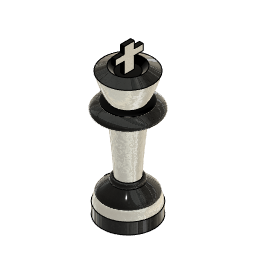
king_chess_piece (Autodesk Fusion 360 design; units mm, degrees)
Autodesk Fusion 360 part; units mm, degrees
sketch "Sketch2" plane through (0, 0, 0) normal (0, 1, 0) x (1, 0, 0)
  line L0 (0, 0) -> (-7, 0)
  line L1 (-7, 0) -> (-7, 3)
  spline S0 degree 5 poles (-7, 3) (-6.9874, 3.0714) (-6.9612, 3.2116) (-6.9188, 3.4141) (-6.856, 3.6679) (-6.7665, 3.9566) (-6.6647, 4.2138) (-6.5496, 4.4365) (-6.4202, 4.6222) (-6.2765, 4.7712) (-6.1194, 4.8856) (-5.9839, 4.9515) (-5.8769, 4.9875) (-5.8034, 5.0055) (-5.766, 5.013) knots 0 0 0 0 0 0 0.1 0.2 0.3 0.4 0.5 0.6 0.7 0.8 0.9 1 1 1 1 1 1
  spline S1 degree 5 poles (-5.766, 5.013) (-5.8491, 5.0166) (-6.0026, 5.0292) (-6.1954, 5.0646) (-6.376, 5.1453) (-6.4673, 5.3049) (-6.4171, 5.5264) (-6.2239, 5.8105) (-5.8977, 6.1528) (-5.4521, 6.5473) (-4.9009, 6.988) (-4.3843, 7.3737) (-3.9572, 7.6802) (-3.6553, 7.8921) (-3.5, 8) knots 0 0 0 0 0 0 0.1 0.2 0.3 0.4 0.5 0.6 0.7 0.8 0.9 1 1 1 1 1 1
  circle A0 centre (-2.9, 8.4) radius 0.7211
  spline S2 degree 5 poles (-2.8459, 9.1191) (-2.8432, 9.2564) (-2.8404, 9.5444) (-2.8435, 10.0169) (-2.8628, 10.7291) (-2.9134, 11.7639) (-2.9922, 12.9521) (-3.0997, 14.2974) (-3.2345, 15.791) (-3.3939, 17.4189) (-3.5752, 19.1663) (-3.736, 20.6501) (-3.8649, 21.8079) (-3.9544, 22.5994) (-4, 23) knots 0 0 0 0 0 0 0.1 0.2 0.3 0.4 0.5 0.6 0.7 0.8 0.9 1 1 1 1 1 1
  spline S3 degree 5 poles (-4, 23) (-4.2423, 23.0544) (-4.708, 23.1636) (-5.3496, 23.3289) (-6.0894, 23.5522) (-6.8078, 23.8366) (-7.2999, 24.1267) (-7.5451, 24.423) (-7.5279, 24.726) (-7.2529, 25.0355) (-6.737, 25.351) (-6.1462, 25.608) (-5.609, 25.8031) (-5.2099, 25.9342) (-5, 26) knots 0 0 0 0 0 0 0.1 0.2 0.3 0.4 0.5 0.6 0.7 0.8 0.9 1 1 1 1 1 1
  spline S4 degree 5 poles (-5, 26) (-5.0554, 26.027) (-5.1592, 26.0801) (-5.2942, 26.1566) (-5.432, 26.2523) (-5.5294, 26.3609) (-5.5464, 26.4575) (-5.4782, 26.5415) (-5.3253, 26.613) (-5.0938, 26.6728) (-4.7909, 26.722) (-4.4968, 26.7537) (-4.249, 26.7734) (-4.0719, 26.7848) (-3.9804, 26.7901) knots 0 0 0 0 0 0 0.1 0.2 0.3 0.4 0.5 0.6 0.7 0.8 0.9 1 1 1 1 1 1
  spline S5 degree 5 poles (-3.9804, 26.7901) (-4.048, 26.9113) (-4.1817, 27.1547) (-4.3776, 27.5219) (-4.6294, 28.0163) (-4.9274, 28.6425) (-5.2072, 29.2778) (-5.4674, 29.9228) (-5.7071, 30.5779) (-5.9271, 31.2427) (-6.1291, 31.9165) (-6.2773, 32.4621) (-6.3815, 32.8747) (-6.4479, 33.1514) (-6.4804, 33.2901) knots 0 0 0 0 0 0 0.1 0.2 0.3 0.4 0.5 0.6 0.7 0.8 0.9 1 1 1 1 1 1
  line L2 (-6.4804, 33.2901) -> (-4, 34.5)
  line L3 (-4, 34.5) -> (-2.7074, 33.3411)
  line L4 (-2.7074, 33.3411) -> (0, 33.3411)
  line L5 (0, 33.3411) -> (0, 0)
  point P0 (-6.5, 4.5)
  point P1 (-6.4, 5.5)
  point P2 (-3, 13)
  point P3 (-7.5, 24.5)
  point P4 (-5.5, 26.5)
  point P5 (-5.4571, 29.9117)
  constraint coincident L0.start L5.end
  constraint horizontal L0
  constraint perpendicular L0 L1
  constraint coincident S1.end A0
  constraint coincident A0 S2.start
  constraint horizontal L4
  constraint perpendicular L0 L5
revolve "Revolve1" add sketch "Sketch2" angle 360 about axis through (0, 0, -33.3411) along (0, 0, 1)
sketch "Sketch14" plane through (0, 0, -33.3411) normal (0, 0, -1) x (1, 0, 0)
  circle A0 centre (0, 0) radius 2.7074
  line L0 (-0.5, 0) -> (-0.5, 1.2)
  line L1 (-0.5, 1.2) -> (0.5, 1.2)
  line L2 (0.5, 1.2) -> (0.5, -1.5)
  line L3 (0.5, -1.5) -> (-0.5, -1.5)
  line L4 (-0.5, -1.5) -> (-0.5, 0)
  constraint vertical L0
  constraint perpendicular L0 L1
  constraint perpendicular L1 L2
  constraint perpendicular L2 L3
  constraint perpendicular L3 L4
extrude "Extrude1" add sketch "Sketch14" along normal blind 6.6 contours L0 L1 L2 L3 L4
sketch "Sketch15" plane through (0, 1.5, 0) normal (0, 1, 0) x (-1, 0, 0)
  line L0 (0.5, -33.3411) -> (-0.5, -33.3411)
  line L1 (-0.5, -33.3411) -> (-0.5, -39.9411)
  line L2 (-0.5, -39.9411) -> (0.5, -39.9411)
  line L3 (0.5, -39.9411) -> (0.5, -33.3411)
  line L4 (0.5, -38.1) -> (-0.5, -38.1)
  line L5 (-0.5, -38.1) -> (-0.5, -36.5)
  line L6 (0.5, -36.5) -> (0.5, -38.1)
  line L7 (0.5, -36.5) -> (-0.5, -36.5)
  constraint coincident L3 L4.start
  constraint coincident L1 L4.end
  constraint perpendicular L1 L4
  constraint coincident L1 L5.end
  constraint coincident L3 L6.start
  constraint perpendicular L4 L6
  constraint perpendicular L5 L7
extrude "Extrude2" add sketch "Sketch15" along normal blind 2.4 contours L1 L3 L4 L5 L6 L7
sketch "Sketch16" plane through (0, -1.2, 0) normal (0, -1, 0) x (1, 0, 0)
  line L0 (0.5, -33.3411) -> (-0.5, -33.3411)
  line L1 (-0.5, -33.3411) -> (-0.5, -39.9411)
  line L2 (-0.5, -39.9411) -> (0.5, -39.9411)
  line L3 (0.5, -39.9411) -> (0.5, -33.3411)
  line L4 (0.5, -38.1) -> (-0.5, -38.1)
  line L5 (-0.5, -36.5) -> (0.5, -36.5)
  constraint coincident L3 L4.start
  constraint coincident L1 L4.end
  constraint perpendicular L1 L4
  constraint coincident L1 L5.start
  constraint coincident L3 L5.end
  constraint perpendicular L3 L5
extrude "Extrude3" add sketch "Sketch16" along normal blind 2.4 contours L1 L3 L4 L5
move_body "Move1" bodies 1 to x (1, 0, 0) y (0, -1, 0) z (0, 0, -1) at (3.1263, -15.0902, 5.7131)
move_body "Move2" bodies 1 to x (1, 0, 0) y (0, 1, 0) z (0, 0, 1) at (0, 0, -5)
